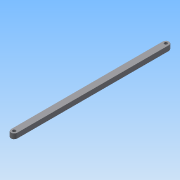
# Autodesk Inventor part: 4
Saved by Autodesk Inventor 2015 (Build 190159000, 159)
## iProperties
Created: 2018-05-07
Part Number: 4
Material: 一般
Document SubType Name: Modeling
Designer: 王博聖
Density: 1 g/cm^3
Appearance: 預設
Author: 王博聖
Autodesk Inventor part; units mm, degrees
ref_plane "YZ Plane" through (0, 0, 0) normal (1, 0, 0) x (0, 1, 0)
ref_plane "XZ Plane" through (0, 0, 0) normal (0, 1, 0) x (-1, 0, 0)
ref_plane "XY Plane" through (0, 0, 0) normal (0, 0, 1) x (1, 0, 0)
sketch "草圖1" plane through (0, 0, 0) normal (0, 0, 1) x (1, 0, 0)
  line L0 (0, 0) -> (0, 60.67) construction
  line L1 (1.25, 0) -> (1.25, 60.67)
  line L2 (-1.25, 60.67) -> (-1.25, 0)
  arc A0 (-1.25, 0) -> (1.25, 0) centre (0, 0) ccw
  arc A1 (1.25, 60.67) -> (-1.25, 60.67) centre (0, 60.67) ccw
  circle A2 centre (0, 0) radius 0.625
  circle A3 centre (0, 60.67) radius 0.625
  point P0 (0, 30.335)
  dimension "d0" = 60.67
  dimension "d1" = 2.5
  dimension "d2" = 1.25
  dimension "d3" = 1.25
  constraints: 8 end point, 4 centre point, 4 point on circle, 4 tangent, 2 coincident, 1 midpoint, 1 parallel, 1 vertical
  measures "d0" distance of L0.start L0.end
  measures "d1" diameter of A1
  measures "d2" diameter of A2
  measures "d3" diameter of A3
extrude "擠出1" add sketch "草圖1" along normal blind 2
